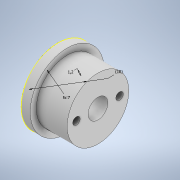
# Autodesk Inventor part: Capston_Tensioning
Saved by Autodesk Inventor 2022 (Build 260153000, 153)
## iProperties
Created: 2023-07-19
Part Number: Capston_Tensioning
Material: Generisch
Document SubType Name: Modeling
Designer: aewalder
Density: 1 g/cm^3
Appearance: Vorgabe
Author: aewalder
Autodesk Inventor part; units mm, degrees
ref_plane "YZ Plane" through (0, 0, 0) normal (1, 0, 0) x (0, 1, 0)
ref_plane "XZ Plane" through (0, 0, 0) normal (0, 1, 0) x (-1, 0, 0)
ref_plane "XY Plane" through (0, 0, 0) normal (0, 0, 1) x (1, 0, 0)
sketch "Sketch1" plane through (0, 0, 0) normal (0, 0, 1) x (1, 0, 0)
  line L0 (0, 0) -> (0, 6)
  line L1 (0, 6) -> (1.5, 6)
  line L2 (1.5, 6) -> (1.5, 5)
  line L3 (1.5, 5) -> (6.5, 5)
  line L4 (6.5, 5) -> (6.5, 0)
  line L5 (6.5, 0) -> (0, 0)
  dimension "d0" = 10
  dimension "d1" = 12
  dimension "d2" = 1.5
  dimension "d17" = 5
  constraints: 12 end point, 5 perpendicular, 1 vertical
  measures "d0" diameter of L3 L5
  measures "d1" diameter of L1 L5
  measures "d2" distance between parallel lines of L0 L2
  measures "d17" distance between parallel lines of L2 L4
revolve "Revolution1" add sketch "Sketch1" angle 360 about axis through (6.5, 0, 0) along (-1, 0, 0)
sketch "Sketch2" plane through (0, 0, 0) normal (-1, 0, 0) x (0, 0, 1)
  circle A0 centre (0, 0) radius 6 projected
  circle A1 centre (-3.5, 0) radius 0.6
  circle A2 centre (3.5, 0) radius 0.6
  line L0 (-3.5, 0) -> (3.5, 0) construction
  circle A3 centre (0, 0) radius 3.5 construction
  circle A4 centre (0, 0) radius 5 construction
  point P0 (0, 0)
  dimension "d6" = 7
  dimension "d5" = 1.2
  dimension "d7" = 10
  constraints: 3 coincident, 2 centre point, 2 end point, 1 equal radius, 1 horizontal, 1 horizontal alignment, 1 midpoint, 2 other
  measures "d5" diameter of A1
  measures "d7" diameter of A4
extrude "Extrusion1" cut sketch "Sketch2" against normal through all contours A1 | A2
hole "Hole1" at (0, 0, 0) direction (1, 0, 0) diameter 3.2 depth 25 clearance for "Zylinderschraube mit Schlitz DIN 84" size "M3" standard "DIN"
sketch "Sketch3" plane through (0, 0, 0) normal (0, 0, 1) x (1, 0, 0)
  circle A0 centre (2.3333, -3.5) radius 0.5
  line L0 (1.5, -5) -> (6.5, -5) construction
  line L1 (1.5, 5) -> (6.5, 5) construction
  line L2 (-1.3, 0) -> (7.8, 0) construction
  line L3 (1.5, -5) -> (6.5, -5) construction
  line L4 (4, -5) -> (4, 5) construction
  line L5 (1.5, 5) -> (6.5, 5) construction
  point P0 (0, 0)
  dimension "d18" = 1
  dimension "d19" = 3.5
  dimension "d22" = 2.5
  dimension "d23" = 1.6667
  constraints: 2 end point, 2 midpoint, 1 centre point
  measures "d18" diameter of A0
  measures "d19" distance from line of L2 A0.centre
  measures "d22" distance from line of L0.start L4
  measures "d23" distance from line of A0.centre L4
extrude "Extrusion2" cut sketch "Sketch3" along normal through all both and the other way through all
equation "\"d23\" = 0.666667 * d22"
body "Solid1"
